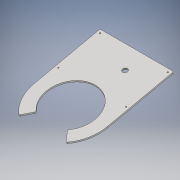
# Autodesk Inventor part: Lock Base
Saved by Autodesk Inventor 2018 (Build 220112000, 112)
## iProperties
Created: 2018-03-09
Part Number: Lock Base
Material: Generic
Document SubType Name: Modeling
Designer: me1160683
Density: 1 g/cm^3
Appearance: Default
Mass: 58.1851 g
Surface Area: 415.375 cm^2
Volume: 58.1851 cm^3
Author: me1160683
Autodesk Inventor part; units mm, degrees
ref_plane "YZ Plane" through (0, 0, 0) normal (1, 0, 0) x (0, 1, 0)
ref_plane "XZ Plane" through (0, 0, 0) normal (0, 1, 0) x (-1, 0, 0)
sketch "Sketch1" plane through (0, 0, 0) normal (0, 0, 1) x (1, 0, 0)
  line L0 (-75, 67.0488) -> (75, 67.0488)
  arc A0 (-75, -67.9512) -> (-48.2091, -125.4046) centre (0, -67.9512) ccw
  arc A1 (48.2091, -125.4046) -> (75, -67.9512) centre (0, -67.9512) ccw
  arc A2 (32.1394, -106.2534) -> (-32.1394, -106.2534) centre (0, -67.9512) ccw
  line L1 (-48.2091, -125.4046) -> (-32.1394, -106.2534) construction
  line L2 (-32.1394, -106.2534) -> (0, -67.9512) construction
  line L3 (-48.2091, -125.4046) -> (-32.1394, -106.2534) construction
  line L4 (75, -67.9512) -> (75, 67.0488)
  line L5 (-75, -67.9512) -> (-75, 67.0488)
  line L6 (0, -67.9512) -> (0, -148.7803) construction
  line L7 (-32.1394, -106.2534) -> (-48.2091, -125.4046)
  line L8 (48.2091, -125.4046) -> (32.1394, -106.2534)
  point P0 (0, 0)
  dimension "d0" = 150
  dimension "d2" = 135
  dimension "d3" = 135
  dimension "d7" = 135
  dimension "d8" = 50
  dimension "d19" = 75
  dimension "d25" = 75
  dimension "d26" = 0
  dimension "d29" = 50
  dimension "d31" = 50
  dimension "d34" = 40
  dimension "d35" = 40
  constraints: 18 end point, 6 point on circle, 3 centre point, 2 coincident, 2 vertical, 1 horizontal, 1 parallel
  measures "d0" distance of L0.start L0.end
  measures "d2" distance of L0.end L4.start
  measures "d3" distance of L0.start L5.start
  measures "d7" distance from line of L0 A0.centre
  measures "d8" radius of A2
  measures "d19" radius of A0
  measures "d25" radius of A1
  measures "d26" horizontal distance of point (0, 0) A0.centre
extrude "Extrusion1" add sketch "Sketch1" along normal blind 3
sketch "Sketch5" plane through (0, 0, 3) normal (0, 0, 1) x (1, 0, 0)
  arc A0 (32.1394, -106.2534) -> (-32.1394, -106.2534) centre (0, -67.9512) ccw projected
  line L0 (32.1394, -106.2534) -> (48.2091, -125.4046) projected
  line L1 (-48.2091, -125.4046) -> (-32.1394, -106.2534) projected
  arc A1 (37.2817, -112.3818) -> (-37.2817, -112.3818) centre (0, -67.9512) ccw
  arc A2 (32.1394, -106.2534) -> (-32.1394, -106.2534) centre (0, -67.9512) ccw projected
  arc A3 (32.1394, -106.2534) -> (-32.1394, -106.2534) centre (0, -67.9512) ccw
  arc A4 (41.7812, -117.7441) -> (-41.7812, -117.7441) centre (0, -67.9512) ccw
  arc A5 (46.2807, -123.1064) -> (-46.2807, -123.1064) centre (0, -67.9512) ccw
  line L2 (-46.2807, -123.1064) -> (-41.7812, -117.7441)
  line L3 (-37.2817, -112.3818) -> (-32.1394, -106.2534)
  line L4 (32.1394, -106.2534) -> (37.2817, -112.3818)
  line L5 (41.7812, -117.7441) -> (46.2807, -123.1064)
  point P0 (0, 0)
  dimension "d49" = 58
  dimension "d52" = 65
  dimension "d53" = 72
  constraints: 8 end point, 8 point on circle, 6 point on line, 4 centre point, 4 coincident, 4 collinear
  measures "d49" radius of A1
  measures "d52" radius of A4
  measures "d53" radius of A5
extrude "Extrusion3" add sketch "Sketch5" along normal blind 8 contours A0 L1 A1 L0 | A4 L1 A5 L0
sketch "Sketch7" plane through (-48.2091, -125.4046, 3) normal (0.7660444, -0.6427876, 0) x (0, 0, -1)
  line L0 (0, 10) -> (-8, 10) projected
  line L1 (-4.5, 10) -> (0, 10)
  line L2 (0, 10) -> (0, 17) projected
  line L3 (0, 10) -> (0, 17)
  line L4 (0, 17) -> (-4.5, 17)
  line L5 (0, 17) -> (-8, 17) projected
  arc A0 (-4.5, 10) -> (-4.5, 17) centre (-4.5, 13.5) ccw
  line L6 (-19.076, 75) -> (19.2246, 75) construction
  point P0 (3, 127.0537)
  dimension "d58" = 4.5
  dimension "d59" = 0
  dimension "d60" = 0
  dimension "d61" = 3.5
  dimension "d62" = 58
  constraints: 8 end point, 2 collinear, 2 point on circle, 2 point on line, 1 centre point, 1 horizontal
  measures "d58" distance of L0.start L1.start
  measures "d59" horizontal distance of L1.start L4.end
  measures "d60" horizontal distance of A0.centre L1.start
  measures "d61" radius of A0
  measures "d62" distance between parallel lines of L6 L4
revolve "Revolution1" add sketch "Sketch7" angle 280 about axis through (0, -67.9512, 22.076) along (0, 0, -1)
sketch "Sketch18" plane through (0, 0, 0) normal (0, 0, -1) x (-1, 0, 0)
  arc A0 (32.1394, -106.2534) -> (-32.1394, -106.2534) centre (0, -67.9512) ccw projected
  line L0 (32.1394, -106.2534) -> (48.2091, -125.4046) projected
  arc A1 (32.1394, -106.2534) -> (-32.1394, -106.2534) centre (0, -67.9512) ccw
  line L1 (-32.1394, -106.2534) -> (-47.5756, -125.4046)
  line L2 (32.1394, -106.2534) -> (48.2091, -125.4046)
  line L3 (75, 67.0488) -> (-75, 67.0488) projected
  line L4 (-75, 67.0488) -> (-75, -67.9512) projected
  arc A2 (-75, -67.9512) -> (-48.2091, -125.4046) centre (0, -67.9512) ccw projected
  line L5 (-48.2091, -125.4046) -> (-32.1394, -106.2534) projected
  arc A3 (32.1394, -106.2534) -> (-32.1394, -106.2534) centre (0, -67.9512) ccw projected
  line L6 (32.1394, -106.2534) -> (48.2091, -125.4046) projected
  arc A4 (48.2091, -125.4046) -> (75, -67.9512) centre (0, -67.9512) ccw projected
  line L7 (75, -67.9512) -> (75, 67.0488) projected
  arc A5 (-75, -67.9512) -> (-48.2091, -125.4046) centre (0, -67.9512) ccw projected
  line L8 (-75, -67.9512) -> (-75, 67.0488)
  line L9 (75, -67.9512) -> (75, 67.0488) projected
  line L10 (75, 67.0488) -> (75, -67.9512)
  arc A6 (-75, -67.9512) -> (-48.2091, -125.4046) centre (0, -67.9512) ccw
  arc A7 (48.2091, -125.4046) -> (75, -67.9512) centre (0, -67.9512) ccw projected
  arc A8 (48.2091, -125.4046) -> (75, -67.9512) centre (0, -67.9512) ccw
  arc A9 (35.4639, -107.3379) -> (-35.4639, -107.3379) centre (0, -67.9512) ccw
  line L11 (0, -67.9512) -> (35.4639, -107.3379) construction
  line L12 (0, -67.9512) -> (-35.4639, -107.3379) construction
  line L13 (0, -67.9512) -> (0, -163.7516) construction
  arc A10 (46.2807, -123.1064) -> (-46.2807, -123.1064) centre (0, -67.9512) ccw construction
  line L14 (72, -67.9512) -> (72, 64.0488)
  line L15 (72, 64.0488) -> (-72, 64.0488)
  line L16 (-72, 64.0488) -> (-72, -67.9512)
  arc A11 (-72, -67.9512) -> (-48.1774, -121.4576) centre (0, -67.9512) ccw
  arc A12 (48.1774, -121.4576) -> (72, -67.9512) centre (0, -67.9512) ccw
  line L17 (-48.1774, -121.4576) -> (-35.4639, -107.3379)
  line L18 (35.4639, -107.3379) -> (48.1774, -121.4576)
  point P0 (0, 0)
  dimension "d99" = 84
  dimension "d100" = 42
  dimension "d101" = 53
  dimension "d102" = 3
  dimension "d103" = 3
  constraints: 24 end point, 16 point on circle, 6 centre point, 6 coincident, 3 tangent, 3 vertical, 2 perpendicular, 2 point on line, 1 collinear, 1 parallel
  measures "d99" angle of L12 L11
  measures "d101" radius of A9
  measures "d102" distance between parallel lines of L3 L15
  measures "d103" horizontal distance of L3.end L15.end
extrude "Extrusion8" add sketch "Sketch18" against normal blind 53
sketch "Sketch19" plane through (75, -67.9512, 0) normal (1, 0, 0) x (0, 0, -1)
  line L0 (-3, 132) -> (-3, 0) projected
  line L1 (-3, 0) -> (-3, 0) projected
  line L2 (-3, 0) -> (-3, 132) projected
  line L3 (-11, 0) -> (-11, -53.5064) projected
  line L4 (-53, 0) -> (-53, 135) projected
  line L5 (-53, 0) -> (-53, -57.4533) projected
  line L6 (0, -57.4533) -> (-53, -57.4533) projected
  line L7 (-53, 135) -> (-53, -57.4533)
  line L8 (-53, -57.4533) -> (-11, -57.4533)
  line L9 (0, 135) -> (-53, 135) projected
  line L10 (-11, -57.4533) -> (-53, 135)
  point P0 (0, 67.9512)
  dimension "d106" = 0
  constraints: 6 end point, 1 perpendicular, 1 point on line
  measures "d106" horizontal distance of L3.end L8.end
extrude "Extrusion9" cut sketch "Sketch19" against normal blind 150
sketch "Sketch20" plane through (-32.1394, -106.2534, 15.1794) normal (0.7660444, -0.6427876, 0) x (0, 0, -1)
  ellipse E0 centre (7.6794, -11.4625) end of major axis (11.1794, -11.4625) minor radius 3.4979 (7.6794, -14.9604) -> (7.6794, -7.9647) ccw projected
  circle A0 centre (7.6794, -11.4625) radius 3.5
  line L0 (-25.5689, 50.0375) -> (41.9904, 50.0375) construction
  point P0 (15.1794, 102.0537)
  dimension "d109" = 61.5
  constraints: 2 end point, 1 centre point, 1 coincident, 1 horizontal, 2 other
  measures "d109" distance from line of L0 point (7.679, -11.463)
revolve "Revolution4" cut sketch "Sketch20" angle 2 about axis through (0.0241, -67.9225, 40.7483) along (0, 0, -1)
mirror "Mirror3" about plane through (0, 0, 0) normal (1, 0, 0) of "Revolution4"
fillet "Fillet1" radius 2 12 edges at (75, 67.0488, 26.5) (-48.2091, -125.4046, 5.5) (-32.1394, -106.2534, 7.5897) (48.2091, -125.4046, 5.5) (32.1394, -106.2534, 7.5897) (-75, 67.0488, 26.5) (0, 67.0488, 0) (-67.9731, -99.6476, 0) (-75, -0.4512, 0) (67.9731, -99.6476, 0) (75, -0.4512, 0) (0, -17.9512, 0)
sketch "Sketch23" plane through (0, 0, 0) normal (0, 0, -1) x (-1, 0, 0)
  arc A0 (43.4935, -116.2556) -> (-43.4935, -116.2556) centre (0, -67.9512) ccw projected
  line L0 (0, -67.9512) -> (0, -128.8082) construction
  arc A1 (43.4935, -116.2556) -> (-43.4935, -116.2556) centre (0, -67.9512) ccw projected
  line L1 (-56.2917, -100.4512) -> (-50.2295, -96.9512) construction
  line L2 (0, -67.9512) -> (-50.2295, -96.9512) construction
  line L3 (-56.2917, -100.4512) -> (0, -67.9512) construction
  circle A2 centre (-55.0106, -95.6701) radius 3.5 construction
  line L4 (-59.6154, -93.8549) -> (-53.1953, -91.0653) construction
  arc A3 (38.8096, -111.0536) -> (-38.8096, -111.0536) centre (0, -67.9512) ccw construction
  arc A4 (-62.3186, -49.4745) -> (-59.6154, -93.8549) centre (0, -67.9512) ccw construction
  line L5 (0, -67.9512) -> (-62.3186, -49.4745) construction
  line L6 (0, -67.9512) -> (-59.6154, -93.8549) construction
  arc A5 (35.4639, -107.3379) -> (-35.4639, -107.3379) centre (0, -67.9512) ccw construction
  arc A6 (-55.6074, -51.4643) -> (-53.1953, -91.0653) centre (0, -67.9512) ccw construction
  line L7 (0, -67.9512) -> (-55.6074, -51.4643) construction
  line L8 (0, -67.9512) -> (-53.1953, -91.0653) construction
  line L9 (-62.3186, -49.4745) -> (-55.6074, -51.4643)
  arc A7 (-62.3186, -49.4745) -> (-56.2917, -100.4512) centre (0, -67.9512) ccw
  arc A8 (-55.6074, -51.4643) -> (-50.2295, -96.9512) centre (0, -67.9512) ccw
  line L10 (-56.2917, -100.4512) -> (-50.2295, -96.9512)
  point P0 (0, 0)
  dimension "d113" = 7
  dimension "d114" = 60
  dimension "d115" = 7
  dimension "d116" = 7
  dimension "d117" = 40
  dimension "d118" = 40
  constraints: 22 end point, 11 point on circle, 5 centre point, 3 coincident, 3 tangent, 1 collinear, 1 vertical
  measures "d113" distance of L1.start L1.end
  measures "d114" angle of L0 L1
  measures "d115" diameter of A2
  measures "d116" distance of L4.start L4.end
  measures "d117" angle of L5 L6
  measures "d118" angle of L7 L8
extrude "Extrusion10" cut sketch "Sketch23" against normal up to next
sketch "Sketch24" plane through (-73, 67.0488, 53) normal (0, -0.2132164, 0.977005) x (1, 0, 0)
  line L0 (146, 0) -> (0, 0) projected
  ellipse E0 centre (0, -2.0471) end of major axis (0, 0) minor radius 2 (0, 0) -> (-2, -2.0471) ccw projected
  line L1 (-2, -138.1774) -> (-2, -2.0471) projected
  ellipse E1 centre (73, -138.1774) end of major axis (73, -61.4122) minor radius 75 (-2, -138.1774) -> (23.235, -195.609) ccw projected
  ellipse E2 centre (24.562, -194.0775) end of major axis (24.562, -196.1246) minor radius 2 (23.235, -195.609) -> (26.0941, -195.3933) ccw projected
  line L2 (39.5998, -178.9191) -> (26.0941, -195.3933) projected
  ellipse E3 centre (38.0677, -177.6032) end of major axis (38.0677, -175.5562) minor radius 2 (39.5998, -178.9191) -> (39.4112, -176.0869) ccw projected
  ellipse E4 centre (73, -138.1774) end of major axis (73, -189.3542) minor radius 50 (106.5888, -176.0869) -> (39.4112, -176.0869) ccw projected
  ellipse E5 centre (107.9323, -177.6032) end of major axis (107.9323, -175.5562) minor radius 2 (106.5888, -176.0869) -> (106.4002, -178.9191) ccw projected
  line L3 (119.9059, -195.3933) -> (106.4002, -178.9191) projected
  ellipse E6 centre (121.438, -194.0775) end of major axis (121.438, -196.1246) minor radius 2 (119.9059, -195.3933) -> (122.765, -195.609) ccw projected
  ellipse E7 centre (73, -138.1774) end of major axis (73, -61.4122) minor radius 75 (122.765, -195.609) -> (148, -138.1774) ccw projected
  line L4 (148, -2.0471) -> (148, -138.1774) projected
  ellipse E8 centre (146, -2.0471) end of major axis (146, 0) minor radius 2 (148, -2.0471) -> (146, 0) ccw projected
  point P0 (73, -76.8075)
  constraints: 9 other
extrude "Extrusion11" add sketch "Sketch24" along normal blind 3
ref_plane "Work Plane1" through (-73, 67.0488, 53) normal (0, -0.2132164, 0.977005) x (1, 0, 0)
split "Split1" plane through (-73, 67.0488, 53) removes the side toward (0, 0.2132164, -0.977005)
sketch "Sketch25" plane through (-73, 66.4091, 55.931) normal (0, -0.2132164, 0.977005) x (1, 0, 0)
  circle A0 centre (88, -40) radius 5
  line L0 (146, 0) -> (0, 0) projected
  line L1 (148, -138.1774) -> (148, -2.0471) projected
  point P0 (73, -76.8075)
  dimension "d124" = 10
  dimension "d125" = 40
  dimension "d126" = 60
  constraints: 1 centre point
  measures "d124" diameter of A0
  measures "d125" distance from line of L0 A0.centre
  measures "d126" distance from line of A0.centre L1
extrude "Extrusion12" cut sketch "Sketch25" against normal blind 10
sketch "Sketch26" plane through (-73, 66.4091, 55.931) normal (0, -0.2132164, 0.977005) x (1, 0, 0)
  circle A0 centre (4, -6.071) radius 1.25
  circle A1 centre (4, -93.071) radius 1.25
  circle A2 centre (142, -93.071) radius 1.25
  circle A3 centre (142, -6.071) radius 1.25
  line L0 (146, 0) -> (0, 0) projected
  line L1 (-2, -2.0471) -> (-2, -138.1774) projected
  line L2 (148, -138.1774) -> (148, -2.0471) projected
  point P0 (73, -76.8075)
  dimension "d129" = 2.5
  dimension "d130" = 2.5
  dimension "d131" = 2.5
  dimension "d132" = 2.5
  dimension "d133" = 6.071
  dimension "d134" = 6.071
  dimension "d135" = 6
  dimension "d136" = 6
  dimension "d137" = 6
  dimension "d138" = 6
  dimension "d139" = 93.071
  dimension "d140" = 93.071
  constraints: 4 centre point
  measures "d129" diameter of A0
  measures "d130" diameter of A1
  measures "d131" diameter of A2
  measures "d132" diameter of A3
  measures "d133" distance from line of L0 A3.centre
  measures "d134" distance from line of L0 A0.centre
  measures "d135" distance from line of A0.centre L1
  measures "d136" distance from line of L2 A3.centre
  measures "d137" distance from line of L2 A2.centre
  measures "d138" distance from line of L1 A1.centre
  measures "d139" distance from line of L0 A1.centre
  measures "d140" distance from line of L0 A2.centre
extrude "Extrusion13" cut sketch "Sketch26" against normal up to next
body "Solid1"
